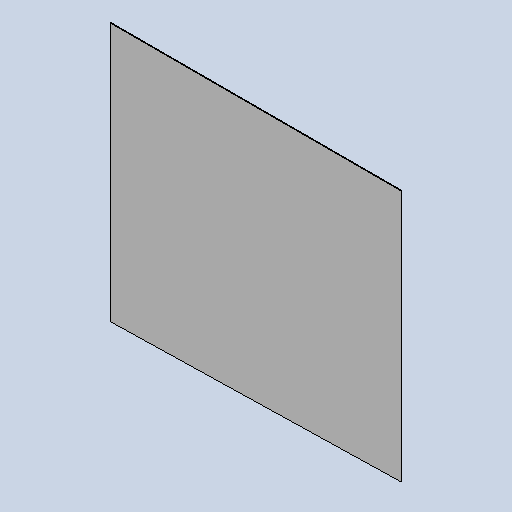
# Autodesk Inventor part: GBK 2111 shield 1
Saved by Autodesk Inventor 2026.2 (Build 302298010, 298A)
## iProperties
Created: 2026-04-17
Part Number: GBK 2111 shield 1
Material: Steel
Document SubType Name: Sheet Metal
Designer: pokla
Stock Number: 2111
Mass: 60330.3 g
Surface Area: 38649.2 cm^2
Volume: 7685.39 cm^3
Density: 7.85 g/cm^3
Sheet Metal Rule: Default_mm
Sheet Metal Width: 1314,662 mm
Sheet Metal Length: 1509,453 mm
Sheet Metal Area: 1984419,668 mm^2
Appearance: Default
Flat Pattern Width: 131.466 cm
Flat Pattern Length: 150.945 cm
Flat Pattern Area: 19844.2 cm^2
Author: admin
Autodesk Inventor part; units mm, degrees
ref_plane "YZ Plane" through (0, 0, 0) normal (1, 0, 0) x (0, 1, 0)
ref_plane "XZ Plane" through (0, 0, 0) normal (0, 1, 0) x (-1, 0, 0)
ref_plane "XY Plane" through (0, 0, 0) normal (0, 0, 1) x (1, 0, 0)
sketch "Sketch1" plane through (0, 0, 0) normal (0, 0, 1) x (1, 0, 0)
  line L0 (740, -745) -> (-740, -745)
  line L1 (-740, -745) -> (-740, 745)
  line L2 (-740, 745) -> (740, 745)
  line L3 (740, 745) -> (740, -745)
  line L4 (740, -745) -> (-740, 745) construction
  line L5 (-740, -745) -> (740, 745) construction
  line L6 (-740, -570) -> (740, -536.4141)
  point P0 (0, 0)
  dimension "d0" = 1480
  dimension "d1" = 1490
  dimension "d3" = 1.3
  dimension "d4" = 175
  dimension "d5" = 1315
  measures "d0" distance of L1.end L2.end
  measures "d1" distance of L0.end L1.end
  measures "d3" angle of L0 L6
  measures "d4" distance of L0.end L6.start
  measures "d5" distance of L6.start L1.end
extrude "Plate1" add sketch "Sketch1" along normal blind 4 contours L6 L1 L2 L3
sketch "Sketch3" plane through (0, 0, 0) normal (0, 0, -1) x (-1, 0, 0)
  line L0 (553.8358, -269.0943) -> (553.8358, -626.7848) construction
  line L1 (553.8358, -626.7848) -> (524.7661, -626.7848) construction
  line L2 (524.7661, -626.7848) -> (524.7661, -269.0943) construction
  line L3 (524.7661, -269.0943) -> (553.8358, -269.0943) construction
  line L4 (710, -489) -> (770, -489) projected
  line L5 (710, -489) -> (710, -485) projected
  line L6 (669.8628, -492.5) -> (669.8628, -589.5) projected
  line L7 (669.8628, -589.5) -> (665.8638, -589.5) projected
  line L8 (710, 7.6667) -> (770, 7.6667) projected
  line L9 (710, 7.6667) -> (710, 11.6667) projected
  line L10 (710, 504.3333) -> (770, 504.3333) projected
  line L11 (710, 504.3333) -> (710, 508.3333) projected
  ellipse E0 centre (669.8628, 745.5) end of major axis (669.8628, 775.5) minor radius 0.6803 (669.8628, 715.5) -> (669.8628, 775.5) ccw projected
  line L12 (669.8628, 715.5) -> (665.8638, 715.5) projected
  ellipse E1 centre (169.7342, 745.5) end of major axis (169.7342, 775.5) minor radius 0.6803 (169.7342, 715.5) -> (169.7342, 775.5) ccw projected
  line L13 (169.7342, 715.5) -> (165.7352, 715.5) projected
  ellipse E2 centre (-330.3944, 745.5) end of major axis (-330.3944, 775.5) minor radius 0.6803 (-330.3944, 715.5) -> (-330.3944, 775.5) ccw projected
  line L14 (-330.3944, 715.5) -> (-334.3934, 715.5) projected
  line L15 (-738.6395, 504.3333) -> (-680, 504.3333) projected
  line L16 (-680, 504.3333) -> (-680, 508.3333) projected
  line L17 (-738.6395, 7.6667) -> (-680, 7.6667) projected
  line L18 (-680, 7.6667) -> (-680, 11.6667) projected
  line L19 (-738.6395, -489) -> (-680, -489) projected
  line L20 (-680, -489) -> (-680, -485) projected
  line L21 (-330.3944, -492.5) -> (-330.3944, -589.5) projected
  line L22 (-330.3944, -589.5) -> (-334.3934, -589.5) projected
  line L23 (169.7342, -492.5) -> (169.7342, -589.5) projected
  line L24 (169.7342, -589.5) -> (165.7352, -589.5) projected
  point P0 (0, 0)
  constraints: 5 other
mark "Mark2"
equation "\"d0\" = Лист_ширина"
equation "\"d1\" = 0.5 * Лист_длина"
equation "\"d2\" = Thickness"
equation "\"BendRadius\" = Thickness"
equation "\"BendReliefWidth\" = Thickness"
equation "\"BendReliefDepth\" = 0.5 * Thickness"
equation "\"CornerReliefSize\" = 4 * Thickness"
equation "\"MinimumRemnant\" = 2 * Thickness"
equation "\"TransitionRadius\" = BendRadius"
equation "\"JacobiRadiusSize\" = BendRadius"
equation "\"GapSize\" = Thickness"
equation "\"Лист_ширина\" = 1480"
equation "\"Лист_длина\" = 2980"
equation "\"Thickness\" = 4"
body "Solid1"
